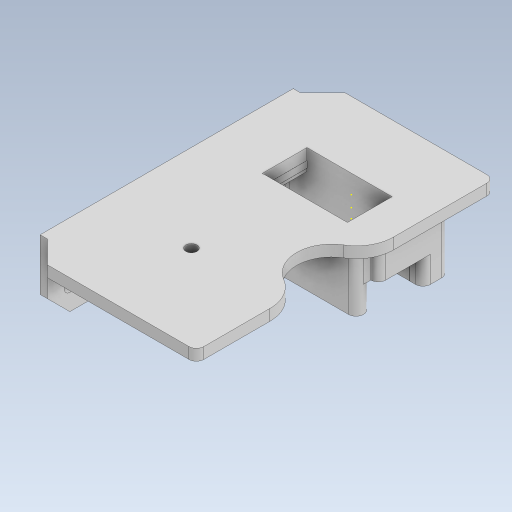
# Autodesk Inventor part: Holder gripper
Saved by Autodesk Inventor 2023.5 (Build 275446000, 446)
## iProperties
Created: 2025-08-31
Part Number: Holder gripper
Material: Generic
Document SubType Name: Modeling
Designer: Naufal K
Density: 1 g/cm^3
Appearance: Default
Mass: 20.7093 g
Surface Area: 133.506 cm^2
Volume: 20.7093 cm^3
Author: Naufal K
## iProperties of the stored document Holder gripper_3DPrint.ipt
Created: 2025-09-05
Part Number: Holder gripper_3DPrint
Material: Generic
Document SubType Name: Modeling
Designer: Guntur
Density: 1 g/cm^3
Appearance: Default
Author: Guntur
Autodesk Inventor part; units mm, degrees
ref_plane "YZ Plane" through (0, 0, 0) normal (1, 0, 0) x (0, 1, 0)
ref_plane "XZ Plane" through (0, 0, 0) normal (0, 1, 0) x (-1, 0, 0)
ref_plane "XY Plane" through (0, 0, 0) normal (0, 0, 1) x (1, 0, 0)
sketch "Sketch3" plane through (0, 0, 0) normal (0, 1, 0) x (-1, 0, 0)
  line L0 (22.7668, 6.9871) -> (-12.2332, 6.9871)
  line L1 (-14.2332, 4.9871) -> (-14.2332, -10.0129)
  line L2 (-12.2332, -12.0129) -> (22.7668, -12.0129)
  line L3 (24.7668, -10.0129) -> (24.7668, 4.9871)
  arc A0 (24.7668, 4.9871) -> (22.7668, 6.9871) centre (22.7668, 4.9871) ccw
  arc A1 (22.7668, -12.0129) -> (24.7668, -10.0129) centre (22.7668, -10.0129) ccw
  arc A2 (-12.2332, 6.9871) -> (-14.2332, 4.9871) centre (-12.2332, 4.9871) ccw
  arc A3 (-14.2332, -10.0129) -> (-12.2332, -12.0129) centre (-12.2332, -10.0129) ccw
  point P0 (0, 0)
  dimension "d4" = 2
  dimension "d7" = 35
  dimension "d10" = 15
  constraints: 8 end point, 8 point on circle, 8 tangent, 4 centre point, 3 equal radius, 2 parallel, 1 horizontal, 1 perpendicular
  measures "d4" radius of A0
  measures "d7" distance of L0.start L0.end
  measures "d10" distance of L1.start L1.end
extrude "Extrusion3" add sketch "Sketch3" along normal blind 14.25
sketch "Sketch4" plane through (0, 14.25, 0) normal (0, 1, 0) x (1, 0, 0)
  point P0 (0, 0)
sketch "Sketch6" plane through (-22.7668, 0, 6.9871) normal (0, 0, 1) x (1, 0, 0)
  line L0 (5.8398, -11.8677) -> (5.8398, -0.1162)
  line L1 (5.8398, -0.1162) -> (1.1747, -0.1162)
  line L2 (1.1747, -0.1162) -> (1.1747, 5.6838)
  line L3 (1.1747, 5.6838) -> (5.8398, 5.6838)
  line L4 (5.8398, 5.6838) -> (5.8398, 12.4478)
  line L5 (5.8398, 12.4478) -> (28.715, 12.4478)
  line L6 (28.715, 12.4478) -> (28.715, 5.6838)
  line L7 (28.715, 5.6838) -> (33.4386, 5.6838)
  line L8 (33.4386, 5.6838) -> (33.4386, -0.1162)
  line L9 (33.4386, -0.1162) -> (28.715, -0.1162)
  line L10 (28.715, -11.8677) -> (5.8398, -11.8677)
  line L11 (28.715, -0.1162) -> (28.715, -11.8677)
  line L12 (5.8579, 12.4478) -> (5.8579, 16.6897)
  line L13 (5.8579, 16.6897) -> (28.715, 16.6897)
  line L14 (28.715, 16.6897) -> (28.715, 12.4478)
  dimension "d33" = 11.0059
  dimension "d38" = 5.8
  constraints: 30 end point, 9 point on line, 8 perpendicular, 1 parallel
  measures "d33" distance of L14.start L6.end
  measures "d38" distance of L7.end L8.end
extrude "Extrusion4" cut sketch "Sketch6" against normal blind 12
sketch "Sketch5" plane through (12.2332, 0, -12.0129) normal (0, 0, -1) x (-1, 0, 0)
  point P0 (12.2332, 0)
sketch "Sketch7" plane through (0, 14.25, 0) normal (0, 1, 0) x (1, 0, 0)
  point P0 (0, 0)
sketch "Sketch8" plane through (-22.7668, 0, 6.9871) normal (0, 0, 1) x (1, 0, 0)
  line L0 (0, 0) -> (0, 14.25) projected
  line L1 (35, 0) -> (0, 0) projected
  line L2 (0, 14.25) -> (35, 14.25)
  line L3 (35, 14.25) -> (35, 0)
  line L4 (35, 0) -> (0, 0)
  line L5 (0, 0) -> (0, 14.25)
  point P0 (22.7668, 0)
  constraints: 8 end point, 2 parallel, 1 horizontal, 1 perpendicular
extrude "Extrusion5" add sketch "Sketch8" along normal blind 4
sketch "Sketch9" plane through (-24.7668, 0, -10.0129) normal (-1, 0, 0) x (0, 0, 1)
  point P0 (10.0129, 0)
sketch "Sketch10" plane through (0, 14.25, 0) normal (0, 1, 0) x (1, 0, 0)
  point P0 (0, 0)
sketch "Sketch15" plane through (0, 14.25, 0) normal (0, 1, 0) x (1, 0, 0)
  line L0 (19.5196, -57.1297) -> (-30.4804, -57.1297)
  line L1 (-30.4804, -57.1297) -> (-30.4804, 22.8703)
  line L2 (-30.4804, 22.8703) -> (19.5196, 22.8703)
  line L3 (15.5136, 22.8703) -> (15.5136, -57.1297)
  line L4 (19.5196, -57.1297) -> (-30.4804, 22.8703) construction
  line L5 (-30.4804, -57.1297) -> (19.5196, 22.8703) construction
  point P0 (0, 0)
  point P1 (-5.4804, -17.1297)
  dimension "d34" = 50
  dimension "d35" = 80
  constraints: 12 end point, 2 midpoint, 2 parallel, 1 horizontal, 1 perpendicular
  measures "d34" distance of L2.end L1.end
  measures "d35" distance of L0.end L1.end
extrude "Extrusion9" add sketch "Sketch15" along normal blind 3
sketch "Sketch16" plane through (0, 14.25, 0) normal (0, -1, 0) x (1, 0, 0)
  line L0 (5.9482, 6.9871) -> (5.9482, -5.0129) projected
  line L1 (-21.5921, 6.9871) -> (-16.927, 6.9871) projected
  line L2 (5.9482, -5.0129) -> (-16.927, -5.0129)
  line L3 (-16.927, -5.0129) -> (-16.927, 6.9871)
  line L4 (-16.927, 6.9871) -> (5.9482, 6.9871)
  line L5 (5.9482, 6.9871) -> (5.9482, -5.0129)
  point P0 (0, 0)
  constraints: 8 end point, 2 parallel, 1 horizontal, 1 perpendicular
extrude "Extrusion10" cut sketch "Sketch16" against normal blind 3
sketch "Sketch17" plane through (-21.5921, 5.6838, -5.0129) normal (0, -1, 0) x (1, 0, 0)
  line L0 (27.5403, 0) -> (32.2639, 0) projected
  line L1 (27.5403, 0) -> (27.5403, 12) projected
  line L2 (32.2639, 0) -> (27.5403, 0)
  line L3 (27.5403, 0) -> (27.5403, 12)
  line L4 (27.5403, 12) -> (32.2639, 12)
  line L5 (32.2639, 12) -> (32.2639, 0)
  line L6 (0, 12) -> (0, 0) projected
  line L7 (4.6651, 0) -> (0, 0)
  line L8 (0, 0) -> (0, 12)
  line L9 (0, 12) -> (4.6651, 12)
  line L10 (4.6651, 12) -> (4.6651, 0)
  point P0 (21.5921, 5.0129)
  constraints: 16 end point, 4 parallel, 2 horizontal, 2 perpendicular
extrude "Extrusion11" cut sketch "Sketch17" against normal blind 6
sketch "Sketch18" plane through (0, 0, 0) normal (0, -1, 0) x (1, 0, 0)
  line L0 (-21.5921, -5.0129) -> (-21.5921, 6.9871) projected
  line L1 (-24.7668, -10.0129) -> (-24.7668, 4.9871) projected
  line L2 (-21.5921, 6.9871) -> (-24.7668, 6.9871)
  line L3 (-24.7668, 6.9871) -> (-24.7668, -4.9898)
  line L4 (-24.7668, -4.9898) -> (-21.5921, -4.9898)
  line L5 (-21.5921, -4.9898) -> (-21.5921, 6.9871)
  line L6 (-21.5921, 6.9871) -> (10.6718, 6.9871) projected
  line L7 (14.2332, 4.9871) -> (14.2332, -10.0129) projected
  line L8 (10.6718, 6.9871) -> (14.2332, 6.9871)
  line L9 (14.2332, 6.9871) -> (14.2332, -4.9898)
  line L10 (14.2332, -4.9898) -> (10.6718, -4.9898)
  line L11 (10.6718, -4.9898) -> (10.6718, 6.9871)
  point P0 (0, 0)
  point P1 (-24.7668, 4.9871)
  constraints: 16 end point, 4 parallel, 3 point on line, 2 horizontal, 2 perpendicular
extrude "Extrusion12" cut sketch "Sketch18" against normal blind 7
fillet "Fillet1" radius 2 4 edges at (12.2332, 3.5, 6.9871) (-22.7668, 3.5, 6.9871) (12.2332, 7.125, 10.9871) (-22.7668, 7.125, 10.9871)
fillet "Fillet2" radius 2 2 edges at (14.2332, 3.5, -4.9898) (-24.7668, 3.5, -4.9898)
sketch "Sketch19" plane through (-21.5921, 11.6838, -5.0129) normal (0, -1, 0) x (1, 0, 0)
  point P0 (21.5921, 5.0129)
chamfer "Chamfer4" distance 6 angle 45 2 edges at (-30.4804, 15.75, 57.1297) (-30.4804, 15.75, -22.8703)
sketch "Sketch20" plane through (0, 17.25, 0) normal (0, 1, 0) x (1, 0, 0)
  point P0 (0, 0)
sketch "Sketch21" plane through (0, 17.25, 0) normal (0, 1, 0) x (1, 0, 0)
  circle A0 centre (-9.0304, -33.9297) radius 1.5
  line L0 (-24.4804, -57.1297) -> (15.5136, -57.1297) projected
  line L1 (-30.4804, 16.8703) -> (-30.4804, -51.1297) projected
  point P0 (0, 0)
  point P1 (13.5196, -57.1297)
  dimension "d50" = 3
  dimension "d51" = 23.2
  dimension "d52" = 21.45
  constraints: 1 centre point
  measures "d50" diameter of A0
  measures "d51" distance from line of A0.centre L0
  measures "d52" distance from line of L1 A0.centre
extrude "Extrusion13" cut sketch "Sketch21" against normal blind 4
sketch "Sketch22" plane through (-30.4804, 14.25, -16.8703) normal (-1, 0, 0) x (0, 0, 1)
  point P0 (16.8703, -14.25)
sketch "Sketch23" plane through (-30.4804, 14.25, -16.8703) normal (-1, 0, 0) x (0, 0, 1)
  point P0 (16.8703, -14.25)
sketch "Sketch24" plane through (-30.4804, 14.25, -16.8703) normal (-1, 0, 0) x (0, 0, 1)
  line L0 (0, 3) -> (68, 3) projected
  line L1 (0, 3) -> (68, 3)
  line L2 (68, 3) -> (68, -16.8762)
  line L3 (68, -16.8762) -> (0, -16.8762)
  line L4 (0, -16.8762) -> (0, 3)
  point P0 (16.8703, -14.25)
  constraints: 8 end point, 2 parallel, 1 horizontal, 1 perpendicular
extrude "Extrusion14" add sketch "Sketch24" along normal blind 2
chamfer "Chamfer5" distance 6 angle 45 2 edges at (-31.4804, -2.6262, 51.1297) (-31.4804, -2.6262, -16.8703)
sketch "Sketch25" plane through (-21.5921, 11.6838, -5.0129) normal (0, -1, 0) x (1, 0, 0)
  circle A0 centre (29.8639, 6.2) radius 1
  line L0 (32.2639, 0.0231) -> (32.2639, 12.0487) projected
  line L1 (32.2639, 0) -> (0, 0) projected
  point P0 (21.5921, 5.0129)
  dimension "d60" = 2
  dimension "d61" = 2.4
  dimension "d62" = 6.2
  constraints: 1 centre point
  measures "d60" diameter of A0
  measures "d61" distance from line of L0 A0.centre
  measures "d62" distance from line of L1 A0.centre
extrude "Extrusion15" cut sketch "Sketch25" against normal blind 4
sketch "Sketch26" plane through (-21.5921, 11.6838, -5.0129) normal (0, -1, 0) x (1, 0, 0)
  circle A0 centre (2.1523, 6) radius 1
  line L0 (32.2639, 0) -> (0, 0) projected
  line L1 (0, 12.1782) -> (0, 0.0231) projected
  point P0 (21.5921, 5.0129)
  dimension "d67" = 6
  dimension "d68" = 2.1523
  constraints: 1 centre point
  measures "d67" distance from line of L0 A0.centre
  measures "d68" distance from line of L1 A0.centre
extrude "Extrusion16" cut sketch "Sketch26" against normal blind 4
fillet "Fillet3" radius 2 2 edges at (15.5136, 15.75, -22.8703) (15.5136, 15.75, 57.1297)
sketch "Sketch27" plane through (0, 14.25, 0) normal (0, -1, 0) x (1, 0, 0)
  line L0 (15.5136, 55.1297) -> (15.5136, -20.8703) projected
  circle A0 centre (15.5136, 20.7647) radius 9.4028
  point P0 (0, 0)
  point P1 (15.5136, 11.3619)
  point P2 (15.5136, 30.1674)
  constraints: 1 centre point, 1 point on line
extrude "Extrusion17" cut sketch "Sketch27" against normal blind 10 contours L0 A0 picked at (12.4022, 20.3869)
fillet "Fillet4" radius 10 2 edges at (15.5136, 15.75, 11.3619) (15.5136, 15.75, 30.1674)
sketch "Sketch28" plane through (-32.4804, 14.25, -16.8703) normal (-1, 0, 0) x (0, 0, 1)
  circle A0 centre (62, -10.8762) radius 1.5
  circle A1 centre (5.8574, -10.8762) radius 1.5
  point P0 (16.8703, -14.25)
  dimension "d73" = 3
  dimension "d74" = 3
  constraints: 2 centre point
  measures "d73" diameter of A0
  measures "d74" diameter of A1
extrude "Extrusion18" cut sketch "Sketch28" against normal blind 10
sketch "Sketch29" plane through (-32.4804, 14.25, -16.8703) normal (-1, 0, 0) x (0, 0, 1)
  circle A0 centre (34, -14.25) radius 1.5
  circle A1 centre (34, -4.25) radius 1.5
  point P0 (16.8703, -14.25)
  dimension "d77" = 3
  dimension "d78" = 3
  dimension "d79" = 10
  constraints: 2 centre point
  measures "d77" diameter of A0
  measures "d78" diameter of A1
  measures "d79" distance of A1.centre A0.centre
extrude "Extrusion19" cut sketch "Sketch29" against normal blind 10
body "Solid2"
